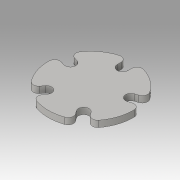
# Autodesk Inventor part: gear wheel
Saved by Autodesk Inventor 2016 (Build 200138000, 138)
## iProperties
Created: 2015-11-24
Part Number: gear wheel
Material: Generic
Document SubType Name: Modeling
Designer: Delta
Density: 1 g/cm^3
Appearance: Default
Author: Delta
Autodesk Inventor part; units mm, degrees
ref_plane "YZ Plane" through (0, 0, 0) normal (1, 0, 0) x (0, 1, 0)
ref_plane "XZ Plane" through (0, 0, 0) normal (0, 1, 0) x (-1, 0, 0)
ref_plane "XY Plane" through (0, 0, 0) normal (0, 0, 1) x (1, 0, 0)
sketch "Sketch1" plane through (0, 0, 0) normal (0, 1, 0) x (-1, 0, 0)
  circle A0 centre (0, 0) radius 76.2
  dimension "d0" = 152.4
  constraints: 1 centre point, 1 coincident
  measures "d0" diameter of A0
extrude "Extrusion1" add sketch "Sketch1" along normal blind 11.43
sketch "Sketch2" plane through (0, 11.43, 0) normal (0, 1, 0) x (1, 0, 0)
  circle A0 centre (0, 0) radius 76.2 projected
  line L0 (0, 76.2) -> (0, 57.15) construction
  arc A1 (-9.5244, 57.0391) -> (9.5244, 57.0391) centre (0, 57.15) ccw
  line L1 (9.5244, 57.0391) -> (9.5244, 75.6024)
  line L2 (-9.5244, 57.0391) -> (-9.5244, 75.6024)
  dimension "d3" = 19.05
  dimension "d4" = 19.05
  constraints: 6 end point, 5 point on circle, 2 parallel, 2 vertical, 1 centre point, 1 coincident
  measures "d3" distance of L0.start L0.end
  measures "d4" diameter of A1
extrude "Extrusion2" cut sketch "Sketch2" against normal through all contours L1 A1 L2 A0 picked at (1.0607, 63.4039)
fillet "Fillet1" radius 9.525 1 edges at (-9.5244, 5.715, -75.6024)
fillet "Fillet2" radius 9.525 1 edges at (9.5244, 5.715, -75.6024)
pattern_circular "Circular Pattern1" count 5 over 360 about axis through (0, -10, 0) along (0, 1, 0) of "Extrusion2", "Fillet1", "Fillet2"
body "Solid1"
